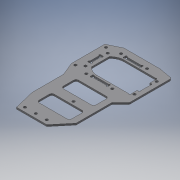
# Autodesk Inventor part: 胴体_サブフレーム_1_3
Saved by Autodesk Inventor 2018 (Build 220112000, 112)
## iProperties
Created: 2016-05-07
Part Number: 胴体_サブフレーム_1_3
Material: GFRP
Document SubType Name: Modeling
Designer: hiroaki
Density: 1.75 g/cm^3
Appearance: 滑らか - 淡い灰色
Mass: 16.0796 g
Surface Area: 112.799 cm^2
Volume: 9.18834 cm^3
d0: 1.000 ul
d2: 2.100 mm
d3: 2.000 mm
d4: 0.00 deg
d7: 8.000 mm
d9: 39.000 mm
d48: 3.000 mm
Author: hiroaki
Autodesk Inventor part; units mm, degrees
ref_plane "YZ Plane" through (0, 0, 0) normal (1, 0, 0) x (0, 1, 0)
ref_plane "XZ Plane" through (0, 0, 0) normal (0, 1, 0) x (-1, 0, 0)
ref_plane "XY Plane" through (0, 0, 0) normal (0, 0, 1) x (1, 0, 0)
derived "胴体_基礎_1_3.ipt"
sketch "スケッチ1" plane through (0, 0, 0) normal (0, 0, 1) x (1, 0, 0)
  circle A0 centre (-13, 0) radius 1.55 projected
  circle A1 centre (13, 0) radius 1.55 projected
  line L0 (0, 0) -> (0, -11.5097) construction
  line L1 (-24, 57.0251) -> (-24, -5) projected
  line L2 (-24, -5) -> (28, -5) projected
  line L3 (-24, 57.0251) -> (-30.5, 72.9658) projected
  line L4 (-30.5, 72.9658) -> (-30.5, 112.7596) projected
  line L5 (-30.5, 112.7596) -> (-15, 120.25) projected
  line L6 (-15, 120.25) -> (28, 120.25) projected
  circle A2 centre (-3, 92) radius 11 construction
  line L7 (-15, 102.583) -> (-15, 81.417) construction
  line L8 (-3, 108) -> (36.5, 108) construction
  line L9 (36.5, 108) -> (36.5, 76) construction
  line L10 (36.5, 76) -> (-3, 76) construction
  arc A3 (-3, 108) -> (-15, 102.583) centre (-3, 92) ccw construction
  arc A4 (-15, 81.417) -> (-3, 76) centre (-3, 92) ccw construction
  line L11 (28, -5) -> (28, 73.75) projected
  line L12 (28, 73.75) -> (28, 120.25) construction
  line L13 (-2, 105.5) -> (25, 105.5) construction
  line L14 (25, 105.5) -> (25, 78.5) construction
  line L15 (25, 78.5) -> (-2, 78.5) construction
  line L16 (-2, 78.5) -> (-2, 105.5) construction
  circle A5 centre (-2, 105.5) radius 1.35 projected
  circle A6 centre (25, 105.5) radius 1.35 projected
  circle A7 centre (25, 78.5) radius 1.35 projected
  circle A8 centre (-2, 78.5) radius 1.35 projected
  circle A9 centre (-3, 92) radius 5.05 projected
  line L17 (-15, 110.25) -> (36.5, 110.25) construction
  line L18 (36.5, 110.25) -> (36.5, 73.75) construction
  line L19 (36.5, 73.75) -> (-15, 73.75) construction
  line L20 (-15, 73.75) -> (-15, 110.25) construction
  circle A10 centre (21.25, 92) radius 1.2 projected
  circle A11 centre (-3, 116.25) radius 1.2 projected
  circle A12 centre (-27.25, 92) radius 1.2 projected
  circle A13 centre (-3, 67.75) radius 1.2 projected
  line L21 (-6, 115.25) -> (15, 115.25) construction
  line L22 (15, 115.25) -> (15, 110.25) construction
  line L23 (15, 110.25) -> (-6, 110.25) construction
  line L24 (-6, 110.25) -> (-6, 115.25) construction
  circle A14 centre (-11, 112.75) radius 1.55 projected
  circle A15 centre (20, 112.75) radius 1.55 projected
  circle A16 centre (-11, 112.75) radius 7.5 construction
  circle A17 centre (-11, 71.25) radius 1.55 projected
  circle A18 centre (20, 71.25) radius 1.55 projected
  line L25 (-15, 92) -> (36.5, 92) construction
  line L26 (-6, 73.75) -> (15, 73.75) construction
  line L27 (15, 73.75) -> (15, 68.75) construction
  line L28 (15, 68.75) -> (-6, 68.75) construction
  line L29 (-6, 68.75) -> (-6, 73.75) construction
  line L30 (-15, 115.25) -> (24, 115.25) construction
  line L31 (24, 115.25) -> (24, 110.25) construction
  line L32 (24, 110.25) -> (-15, 110.25) construction
  line L33 (-15, 110.25) -> (-15, 115.25) construction
  circle A19 centre (-5, 112.8) radius 1.05
  circle A20 centre (14, 112.8) radius 1.05
  circle A21 centre (14.0984, 110.6437) radius 1.05
  circle A22 centre (-20, 50) radius 1.55 projected
  circle A23 centre (-20, 20) radius 1.55 projected
  circle A24 centre (10, 35) radius 1.55 projected
  line L34 (-39.5, 5) -> (35.9852, 5) construction
  line L35 (35.9852, 5) -> (35.9852, -12.9857) construction
  line L36 (35.9852, -12.9857) -> (-39.5, -12.9857) construction
  line L37 (-39.5, -12.9857) -> (-39.5, 5) construction
  line L38 (-12, 60) -> (27, 60)
  line L39 (27, 60) -> (27, 42)
  line L40 (27, 42) -> (-12, 42)
  line L41 (-12, 42) -> (-12, 60)
  line L42 (-12, 31) -> (27, 31)
  line L43 (27, 31) -> (27, 13)
  line L44 (27, 13) -> (-12, 13)
  line L45 (-12, 13) -> (-12, 31)
  line L46 (-15.05, 102.6019) -> (-15.05, 81.3981)
  arc A25 (-15.05, 81.3981) -> (-3, 75.95) centre (-3, 92) ccw
  line L47 (-3, 75.95) -> (36.55, 75.95) construction
  line L48 (36.55, 75.95) -> (36.55, 108.05)
  line L49 (36.55, 108.05) -> (-3, 108.05) construction
  arc A26 (-3, 108.05) -> (-15.05, 102.6019) centre (-3, 92) ccw
  line L50 (28, 120.25) -> (28, 108.05)
  line L51 (28, 108.05) -> (-3, 108.05)
  line L52 (-3, 75.95) -> (28, 75.95)
  line L53 (28, 75.95) -> (28, 73.75)
  line L54 (-15.5, 120.25) -> (24.5, 120.25) construction
  line L55 (4.5, 115.25) -> (4.5, 113.2) construction
  line L56 (-6.05, 112.8) -> (15.05, 112.8)
  line L57 (15.05, 112.8) -> (15.05, 110.2)
  line L58 (15.05, 110.2) -> (-6.05, 110.2)
  line L59 (-6.05, 110.2) -> (-6.05, 112.8)
  circle A27 centre (-5.0984, 110.6437) radius 1.05
  line L60 (-5.0984, 110.6437) -> (-6.05, 110.2) construction
  line L61 (-6.05, 71.2) -> (15.05, 71.2)
  line L62 (15.05, 71.2) -> (15.05, 73.8)
  line L63 (15.05, 73.8) -> (-6.05, 73.8)
  line L64 (-6.05, 73.8) -> (-6.05, 71.2)
  circle A28 centre (-5, 71.2) radius 1.05
  circle A29 centre (14, 71.2) radius 1.05
  circle A30 centre (14.0984, 73.3563) radius 1.05
  circle A31 centre (-5.0984, 73.3563) radius 1.05
  line L65 (-11, 112.75) -> (-11, 71.25) construction
  circle A32 centre (-19.5, 105.25) radius 1.55 projected
  circle A33 centre (-19.5, 78.75) radius 1.55 projected
  line L66 (-22, 99.5) -> (-17, 99.5) construction
  line L67 (-17, 99.5) -> (-17, 84.5) construction
  line L68 (-17, 84.5) -> (-22, 84.5) construction
  line L69 (-22, 84.5) -> (-22, 99.5) construction
  circle A34 centre (-19.5, 100.55) radius 1.05 construction
  line L70 (-22.05, 99.55) -> (-19.45, 99.55)
  line L71 (-19.45, 99.55) -> (-19.45, 84.45)
  line L72 (-19.45, 84.45) -> (-22.05, 84.45)
  line L73 (-22.05, 84.45) -> (-22.05, 99.55)
  circle A35 centre (-22.05, 98.5) radius 1.05
  circle A36 centre (-19.45, 98.5) radius 1.05
  circle A37 centre (-22.05, 85.5) radius 1.05
  circle A38 centre (-19.45, 85.5) radius 1.05
  circle A39 centre (-26.5, 110.25) radius 1.55 projected
  circle A40 centre (-26.5, 73.75) radius 1.55 projected
  circle A41 centre (-26.5, 110.25) radius 4 construction
  circle A42 centre (-26.5, 73.75) radius 4 construction
  circle A43 centre (0, 0) radius 1.55 projected
  point P0 (25, 92)
  point P1 (-6, 112.75)
  point P2 (4.5, 120.25)
  point P3 (-19.5, 99.5)
  dimension "d2" = 2.1
  dimension "d82" = 2.1
  dimension "d7" = 8
  dimension "d9" = 39
  dimension "d54" = 0.05
  dimension "d72" = 0.05
  dimension "d73" = 0.05
  dimension "d74" = 2.6
  dimension "d75" = 25
  dimension "d78" = 0.05
  dimension "d79" = 0.05
  dimension "d80" = 0.05
  dimension "d81" = 0.05
  dimension "d101" = 8
  dimension "d102" = 18
  dimension "d103" = 7
  constraints: 64 end point, 10 parallel, 9 point on line, 9 symmetric about line, 8 centre point, 8 vertical alignment, 7 perpendicular, 6 horizontal, 5 equal radius, 4 point on circle, 3 collinear, 2 midpoint, 1 horizontal alignment, 21 other
  measures "d7" distance from line of A22.centre L41
  measures "d9" distance of L38.start L38.end
  measures "d54" radial gap between concentric circles of A26 A3
  measures "d72" distance between parallel lines of L59 L24
  measures "d73" distance between parallel lines of L58 L32
  measures "d74" distance of L58.end L56.start
  measures "d75" angle of L58 L60
  measures "d78" distance from line of L71 A32.centre
  measures "d79" distance between parallel lines of L70 L66
  measures "d80" distance between parallel lines of L72 L68
  measures "d81" distance between parallel lines of L73 L69
  measures "d101" distance between parallel lines of L34 L44
  measures "d102" distance of L44.end L42.start
  measures "d103" distance from line of A24.centre L40
extrude "押し出し1" add sketch "スケッチ1" along normal blind 2 contours L3 L4 L5 L6 L50 L51 A26 L46 A25 L52 L53 L11 L2 L1 | A11 | A12 | A13 | A22 | A23
fillet "フィレット1" radius 3 8 edges at (-12, 60, 1) (-12, 42, 1) (27, 60, 1) (27, 42, 1) (-12, 31, 1) (-12, 13, 1) (27, 31, 1) (27, 13, 1)
sketch "スケッチ5" plane through (-15, 120.25, 2) normal (0, 0, 1) x (1, 0, 0)
  line L0 (43, -125.25) -> (43, -44.3) projected
  line L1 (-0.05, -38.8519) -> (-0.05, -17.6481) projected
  line L2 (43, -12.2) -> (43, 0) projected
  line L3 (43, 0) -> (59.5, -2.9094)
  line L4 (59.5, -2.9094) -> (59.5, -52.9094)
  line L5 (43, -44.3) -> (50.0151, -44.3)
  line L6 (50.0151, -12.2) -> (43, -12.2)
  circle A0 centre (-4.5, -41.5) radius 1.55 projected
  circle A1 centre (-4.5, -15) radius 1.55 projected
  arc A2 (-0.05, -38.8519) -> (12, -44.3) centre (12, -28.25) ccw projected
  line L7 (51.5, -13.6849) -> (51.5, -20.7)
  line L8 (51.5, -42.8151) -> (51.5, -35.8)
  line L9 (51.5, -20.7) -> (52.5651, -20.7)
  line L10 (52.5651, -35.8) -> (51.5, -35.8)
  line L11 (54.05, -22.1849) -> (54.05, -34.3151)
  arc A3 (54.05, -22.1849) -> (52.5651, -20.7) centre (53.3075, -21.4425) ccw
  circle A4 centre (53.3075, -21.4425) radius 1.05 construction
  line L12 (52.5651, -20.7) -> (54.05, -20.7) construction
  line L13 (54.05, -20.7) -> (54.05, -22.1849) construction
  line L14 (53.3075, -21.4425) -> (54.05, -20.7) construction
  arc A5 (52.5651, -35.8) -> (54.05, -34.3151) centre (53.3075, -35.0575) ccw
  line L15 (12, -28.25) -> (-0.05, -28.25) construction
  circle A6 centre (54, -15) radius 1.55
  circle A7 centre (54, -41.5) radius 1.55
  arc A8 (51.5, -13.6849) -> (50.0151, -12.2) centre (50.7575, -12.9425) ccw
  line L16 (51.5, -13.6849) -> (51.5, -12.2) construction
  line L17 (51.5, -12.2) -> (50.0151, -12.2) construction
  arc A9 (50.0151, -44.3) -> (51.5, -42.8151) centre (50.7575, -43.5575) ccw
  line L18 (51.5, -42.8151) -> (51.5, -44.3) construction
  line L19 (50.0151, -44.3) -> (51.5, -44.3) construction
  line L20 (43, 0) -> (0, 0) projected
  line L21 (-9, -63.2249) -> (-9, -125.25) projected
  line L22 (59.5, -52.9094) -> (49, -63.4094)
  line L23 (49, -63.4094) -> (49, -125.25)
  line L24 (43, -125.25) -> (49, -125.25)
  point P0 (15, -120.25)
  point P1 (-4.45, -35.8)
  point P2 (-4.45, -20.7)
  dimension "d85" = 2.1
  dimension "d84" = 45
  dimension "d89" = 39.5
  dimension "d90" = 2.55
  dimension "d91" = 2.5
  dimension "d92" = 1.05
  dimension "d93" = 170
  dimension "d97" = 8
  dimension "d104" = 45
  dimension "d105" = 58
  dimension "d106" = 50
  constraints: 40 end point, 10 point on circle, 7 horizontal, 6 centre point, 6 vertical, 4 equal radius, 4 horizontal alignment, 3 perpendicular, 2 collinear, 2 vertical alignment, 1 coincident, 1 midpoint, 1 symmetric about line, 5 other
  measures "d84" angle of L12 L14
  measures "d89" distance from line of L15.start L7
  measures "d90" distance between parallel lines of L11 L7
  measures "d91" distance from line of L7 A6.centre
  measures "d92" radius of A8
  measures "d93" angle of L20 L3
  measures "d97" distance between parallel lines of L4 L7
  measures "d104" angle of L22 L5
  measures "d105" distance between parallel lines of L21 L23
  measures "d106" distance of L3.end L4.end
extrude "押し出し4" add sketch "スケッチ5" against normal blind 2 contours L0 L5 A9 L8 L10 A5 L11 A3 L9 L7 A8 L6 L2 L3 L4 L22 L23 L24
fillet "フィレット2" radius 2 8 edges at (28, 120.25, 1) (44.5, 117.3406, 1) (44.5, 67.3406, 1) (36.5, 77.4349, 1) (35.0151, 108.05, 1) (35.0151, 75.95, 1) (36.5, 106.5651, 1) (34, 56.8406, 1)
sketch "スケッチ6" plane through (-24, -5, 2) normal (0, 0, 1) x (1, 0, 0)
  line L0 (8.95, 86.3981) -> (8.95, 107.6019) projected
  arc A0 (21, 113.05) -> (8.95, 107.6019) centre (21, 97) ccw projected
  circle A1 centre (9.9016, 107.1581) radius 1.05
  line L1 (8.95, 107.6019) -> (21, 113.05) construction
  line L2 (9.9016, 107.1581) -> (8.95, 107.6019) construction
  circle A2 centre (9.9016, 86.8419) radius 1.05
  line L3 (21, 97) -> (8.95, 97) construction
  line L4 (0, 62.0251) -> (0, 0) projected
  line L5 (0, 0) -> (58, 0) projected
  line L6 (58, 0) -> (58, 61.0122) projected
  line L7 (0, 24.5177) -> (6, 0)
  line L8 (58, 19.0681) -> (42, 0)
  circle A3 centre (11, 5) radius 1.55 projected
  circle A4 centre (37, 5) radius 1.55 projected
  circle A5 centre (4, 25) radius 1.55 projected
  line L9 (6, 0) -> (42, 0) construction
  line L10 (42, 0) -> (42, 10) construction
  line L11 (42, 10) -> (6, 10) construction
  line L12 (6, 10) -> (6, 0) construction
  circle A6 centre (4, 25) radius 4 construction
  line L13 (42, 10) -> (58, 29.0681) construction
  dimension "d107" = 2.1
  dimension "d108" = 65
  dimension "d111" = 10
  dimension "d112" = 5
  dimension "d113" = 5
  dimension "d114" = 130
  constraints: 20 end point, 5 point on line, 3 parallel, 2 tangent, 1 centre point, 1 coincident, 1 horizontal, 1 midpoint, 1 perpendicular, 1 symmetric about line, 6 other
  measures "d108" angle of L0 L2
  measures "d111" distance between parallel lines of L9 L11
  measures "d112" distance from line of A3.centre L12
  measures "d113" distance from line of L10 A4.centre
  measures "d114" angle of L11 L13
extrude "押し出し5" cut sketch "スケッチ6" against normal blind 10 contours A2 L0 | L0 A2 | A1 L0 | L0 A0 A1 | A1 A0 | L7 L5 L4 | L8 L6 L5
